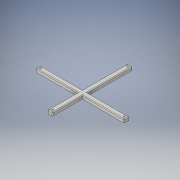
# Autodesk Inventor part: BatteryCrossStrap
Saved by Autodesk Inventor 2016 (Build 200138000, 138)
## iProperties
Created: 2015-09-14
Part Number: BatteryCrossStrap
Material: Generic
Document SubType Name: Modeling
Designer: lachesis
Density: 1 g/cm^3
Appearance: Default
Author: lachesis
Autodesk Inventor part; units mm, degrees
ref_plane "YZ Plane" through (0, 0, 0) normal (1, 0, 0) x (0, 1, 0)
ref_plane "XZ Plane" through (0, 0, 0) normal (0, 1, 0) x (-1, 0, 0)
ref_plane "XY Plane" through (0, 0, 0) normal (0, 0, 1) x (1, 0, 0)
sketch "Sketch1" plane through (0, 0, 0) normal (0, 1, 0) x (-1, 0, 0)
  line L0 (85.471, 4.7625) -> (-85.471, 4.7625)
  line L1 (-85.471, 4.7625) -> (-85.471, -4.7625)
  line L2 (-85.471, -4.7625) -> (85.471, -4.7625)
  line L3 (85.471, -4.7625) -> (85.471, 4.7625)
  line L4 (4.7625, 62.5475) -> (-4.7625, 62.5475)
  line L5 (-4.7625, 62.5475) -> (-4.7625, -91.6305)
  line L6 (-4.7625, -91.6305) -> (4.7625, -91.6305)
  line L7 (4.7625, -91.6305) -> (4.7625, 62.5475)
  point P0 (0, 0)
  point P1 (0, -4.7625)
  point P2 (85.471, 0)
  point P3 (4.7625, -14.5415)
  point P4 (0, 62.5475)
  dimension "d0" = 9.525
  dimension "d1" = 170.942
  dimension "d2" = 154.178
  dimension "d6" = 57.785
  constraints: 16 end point, 4 midpoint, 4 parallel, 3 perpendicular, 2 horizontal, 2 vertical alignment, 1 horizontal alignment
  measures "d0" distance of L2.end L0.start
  measures "d1" distance of L1.end L2.end
  measures "d2" distance of L6.end L4.start
  measures "d6" distance between parallel lines of L4 L0
extrude "Extrusion1" add sketch "Sketch1" along normal blind 6.35
sketch "Sketch2" plane through (0, 6.35, 0) normal (0, 1, 0) x (1, 0, 0)
  line L0 (4.7625, 91.6305) -> (-4.7625, 91.6305) projected
  line L1 (85.471, -4.7625) -> (85.471, 4.7625) projected
  line L2 (-4.7625, -62.5475) -> (4.7625, -62.5475) projected
  line L3 (-85.471, 4.7625) -> (-85.471, -4.7625) projected
  point P0 (0, 0)
  point P1 (0, 86.9315)
  point P2 (0, -57.8485)
  point P3 (-80.772, 0)
  point P4 (80.772, 0)
  dimension "d7" = 4.699
  dimension "d8" = 4.699
  dimension "d9" = 4.699
  dimension "d10" = 4.699
  constraints: 2 horizontal alignment, 2 vertical alignment
  measures "d7" distance from line of L0 point (0, 86.931)
  measures "d8" distance from line of L1 point (80.772, 0)
  measures "d9" distance from line of L2 point (0, -57.849)
  measures "d10" distance from line of L3 point (-80.772, 0)
hole "Hole1" at (0, 6.35, -86.9315) at (0, 6.35, 57.8485) at (-80.772, 6.35, 0) at (80.772, 6.35, 0) direction (0, -1, 0) diameter 3.302 end through all
fillet "Fillet1" radius 1.27 20 edges at (-45.1168, 6.35, 4.7625) (4.7625, 6.35, 33.655) (-4.7625, 6.35, 33.655) (45.1167, 6.35, 4.7625) (4.7625, 6.35, -48.1965) (-4.7625, 6.35, -48.1965) (-45.1167, 6.35, -4.7625) (45.1168, 6.35, -4.7625) (85.471, 3.175, 4.7625) (85.471, 3.175, -4.7625) (85.471, 6.35, 0) (4.7625, 3.175, 62.5475) (0, 6.35, 62.5475) (-4.7625, 3.175, 62.5475) (-85.471, 3.175, 4.7625) (-85.471, 6.35, 0) (4.7625, 3.175, -91.6305) (0, 6.35, -91.6305) (-4.7625, 3.175, -91.6305) (-85.471, 3.175, -4.7625)
equation "\"d8\" = d7"
equation "\"d9\" = d7"
equation "\"d10\" = d7"
body "Solid1"
